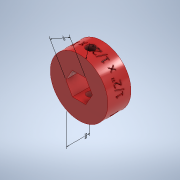
# Autodesk Inventor part: 1_2x1_2x1-1_2 HexBearing
Saved by Autodesk Inventor 2022.2 (Build 262287000, 287)
## iProperties
Created: 2020-11-08
Part Number: 1_2x1_2x1-1_2 HexBearing
Material: PC/ABS Plastic
Document SubType Name: Modeling
Designer: robst
Density: 0.357273 g/cm^3
Appearance: Red
Author: robst
Autodesk Inventor part; units mm, degrees
ref_plane "YZ Plane" through (0, 0, 0) normal (1, 0, 0) x (0, 1, 0)
ref_plane "XZ Plane" through (0, 0, 0) normal (0, 1, 0) x (-1, 0, 0)
ref_plane "XY Plane" through (0, 0, 0) normal (0, 0, 1) x (1, 0, 0)
sketch "Sketch1" plane through (0, 0, 0) normal (0, 0, 1) x (1, 0, 0)
  line L0 (3.6662, 6.35) -> (7.3323, 0)
  line L1 (7.3323, 0) -> (3.6662, -6.35)
  line L2 (3.6662, -6.35) -> (-3.6662, -6.35)
  line L3 (-3.6662, -6.35) -> (-7.3323, 0)
  line L4 (-7.3323, 0) -> (-3.6662, 6.35)
  line L5 (-3.6662, 6.35) -> (3.6662, 6.35)
  circle A0 centre (0, 0) radius 15.875
  circle A1 centre (0, 0) radius 7.3323 construction
  dimension "d0" = 12.7
  dimension "d2" = 31.75
  dimension "d3" = 8.5427
  constraints: 12 end point, 3 coincident, 1 centre point, 1 horizontal, 1 horizontal alignment, 15 other
  measures "d0" distance between parallel lines of L2 L5
  measures "d2" diameter of A0
extrude "Extrusion1" add sketch "Sketch1" against normal blind 12.7
ref_plane "Work Plane1" through (0, 15.875, 0) normal (0, 1, 0) x (-1, 0, 0)
sketch "Sketch2" plane through (0, 15.875, 0) normal (0, 1, 0) x (-1, 0, 0)
  line L0 (0, -6.35) -> (-25.4, -6.35) construction
  line L1 (15.875, 0) -> (-15.875, 0) construction
  line L2 (-22.9639, -8.255) -> (-24.8226, -8.255)
  line L3 (-24.8226, -8.255) -> (-24.8226, -7.866)
  line L4 (-24.8226, -7.866) -> (-24.131, -7.866)
  line L5 (-24.131, -7.866) -> (-24.131, -5.3126)
  line L6 (-24.131, -5.3126) -> (-24.8226, -5.3126)
  line L7 (-24.8226, -5.3126) -> (-24.8226, -4.9637)
  spline S0 degree 2 poles (-24.8226, -4.9637) (-24.4305, -4.9637) (-24.06, -4.7414) (-24.0353, -4.4326) knots 0 0 0 1 2 2 2
  line L8 (-24.0353, -4.4326) -> (-23.6401, -4.4326)
  line L9 (-23.6401, -4.4326) -> (-23.6401, -7.866)
  line L10 (-23.6401, -7.866) -> (-22.9639, -7.866)
  line L11 (-22.9639, -7.866) -> (-22.9639, -8.255)
  line L12 (-20.6792, -4.2752) -> (-22.1705, -9.0825)
  line L13 (-22.1705, -9.0825) -> (-22.6027, -9.0825)
  line L14 (-22.6027, -9.0825) -> (-21.1176, -4.2752)
  line L15 (-21.1176, -4.2752) -> (-20.6792, -4.2752)
  line L16 (-17.9097, -8.255) -> (-20.2593, -8.255)
  line L17 (-20.2593, -8.255) -> (-20.2593, -7.7147)
  spline S1 degree 2 poles (-20.2593, -7.7147) (-20.0061, -7.4769) (-19.5553, -7.0354) (-19.3392, -6.7977) knots 0 0 0 1 2 2 2
  spline S2 degree 2 poles (-19.3392, -6.7977) (-18.9039, -6.3191) (-18.5858, -5.7448) (-18.5858, -5.4392) knots 0 0 0 1 2 2 2
  spline S3 degree 2 poles (-18.5858, -5.4392) (-18.5858, -5.2786) (-18.6846, -5.0378) (-18.7742, -4.9606) knots 0 0 0 1 2 2 2
  spline S4 degree 2 poles (-18.7742, -4.9606) (-18.8637, -4.8834) (-19.0984, -4.8062) (-19.2404, -4.8062) knots 0 0 0 1 2 2 2
  spline S5 degree 2 poles (-19.2404, -4.8062) (-19.3762, -4.8062) (-19.6541, -4.8742) (-19.7807, -4.9267) knots 0 0 0 1 2 2 2
  spline S6 degree 2 poles (-19.7807, -4.9267) (-19.8888, -4.9699) (-20.0895, -5.0934) (-20.1512, -5.1366) knots 0 0 0 1 2 2 2
  line L18 (-20.1512, -5.1366) -> (-20.179, -5.1366)
  line L19 (-20.179, -5.1366) -> (-20.179, -4.5932)
  spline S7 degree 2 poles (-20.179, -4.5932) (-20.0215, -4.516) (-19.4565, -4.3647) (-19.2033, -4.3647) knots 0 0 0 1 2 2 2
  spline S8 degree 2 poles (-19.2033, -4.3647) (-18.6692, -4.3647) (-18.0671, -4.9297) (-18.0671, -5.4114) knots 0 0 0 1 2 2 2
  spline S9 degree 2 poles (-18.0671, -5.4114) (-18.0671, -5.6368) (-18.1721, -6.0135) (-18.2647, -6.174) knots 0 0 0 1 2 2 2
  spline S10 degree 2 poles (-18.2647, -6.174) (-18.3574, -6.3407) (-18.626, -6.668) (-18.7742, -6.8255) knots 0 0 0 1 2 2 2
  spline S11 degree 2 poles (-18.7742, -6.8255) (-19.015, -7.0879) (-19.6047, -7.6498) (-19.7807, -7.8135) knots 0 0 0 1 2 2 2
  line L20 (-19.7807, -7.8135) -> (-17.9097, -7.8135)
  line L21 (-17.9097, -7.8135) -> (-17.9097, -8.255)
  line L22 (-15.8657, -4.2752) -> (-15.9769, -5.7572)
  line L23 (-15.9769, -5.7572) -> (-16.3134, -5.7572)
  line L24 (-16.3134, -5.7572) -> (-16.4246, -4.2752)
  line L25 (-16.4246, -4.2752) -> (-15.8657, -4.2752)
  line L26 (-16.829, -4.2752) -> (-16.9402, -5.7572)
  line L27 (-16.9402, -5.7572) -> (-17.2767, -5.7572)
  line L28 (-17.2767, -5.7572) -> (-17.3879, -4.2752)
  line L29 (-17.3879, -4.2752) -> (-16.829, -4.2752)
  line L30 (-11.3703, -8.255) -> (-11.96, -8.255)
  line L31 (-11.96, -8.255) -> (-12.6547, -7.1805)
  line L32 (-12.6547, -7.1805) -> (-13.3679, -8.255)
  line L33 (-13.3679, -8.255) -> (-13.9144, -8.255)
  line L34 (-13.9144, -8.255) -> (-12.9233, -6.8378)
  line L35 (-12.9233, -6.8378) -> (-13.9052, -5.396)
  line L36 (-13.9052, -5.396) -> (-13.3154, -5.396)
  line L37 (-13.3154, -5.396) -> (-12.6238, -6.4612)
  line L38 (-12.6238, -6.4612) -> (-11.9168, -5.396)
  line L39 (-11.9168, -5.396) -> (-11.3703, -5.396)
  line L40 (-11.3703, -5.396) -> (-12.3552, -6.807)
  line L41 (-12.3552, -6.807) -> (-11.3703, -8.255)
  line L42 (-7.2732, -8.255) -> (-9.1319, -8.255)
  line L43 (-9.1319, -8.255) -> (-9.1319, -7.866)
  line L44 (-9.1319, -7.866) -> (-8.4403, -7.866)
  line L45 (-8.4403, -7.866) -> (-8.4403, -5.3126)
  line L46 (-8.4403, -5.3126) -> (-9.1319, -5.3126)
  line L47 (-9.1319, -5.3126) -> (-9.1319, -4.9637)
  spline S12 degree 2 poles (-9.1319, -4.9637) (-8.7397, -4.9637) (-8.3692, -4.7414) (-8.3445, -4.4326) knots 0 0 0 1 2 2 2
  line L48 (-8.3445, -4.4326) -> (-7.9493, -4.4326)
  line L49 (-7.9493, -4.4326) -> (-7.9493, -7.866)
  line L50 (-7.9493, -7.866) -> (-7.2732, -7.866)
  line L51 (-7.2732, -7.866) -> (-7.2732, -8.255)
  line L52 (-4.9884, -4.2752) -> (-6.4797, -9.0825)
  line L53 (-6.4797, -9.0825) -> (-6.9119, -9.0825)
  line L54 (-6.9119, -9.0825) -> (-5.4268, -4.2752)
  line L55 (-5.4268, -4.2752) -> (-4.9884, -4.2752)
  line L56 (-2.2189, -8.255) -> (-4.5685, -8.255)
  line L57 (-4.5685, -8.255) -> (-4.5685, -7.7147)
  spline S13 degree 2 poles (-4.5685, -7.7147) (-4.3153, -7.4769) (-3.8645, -7.0354) (-3.6484, -6.7977) knots 0 0 0 1 2 2 2
  spline S14 degree 2 poles (-3.6484, -6.7977) (-3.2131, -6.3191) (-2.8951, -5.7448) (-2.8951, -5.4392) knots 0 0 0 1 2 2 2
  spline S15 degree 2 poles (-2.8951, -5.4392) (-2.8951, -5.2786) (-2.9939, -5.0378) (-3.0834, -4.9606) knots 0 0 0 1 2 2 2
  spline S16 degree 2 poles (-3.0834, -4.9606) (-3.1729, -4.8834) (-3.4076, -4.8062) (-3.5496, -4.8062) knots 0 0 0 1 2 2 2
  spline S17 degree 2 poles (-3.5496, -4.8062) (-3.6855, -4.8062) (-3.9633, -4.8742) (-4.0899, -4.9267) knots 0 0 0 1 2 2 2
  spline S18 degree 2 poles (-4.0899, -4.9267) (-4.198, -4.9699) (-4.3987, -5.0934) (-4.4604, -5.1366) knots 0 0 0 1 2 2 2
  line L58 (-4.4604, -5.1366) -> (-4.4882, -5.1366)
  line L59 (-4.4882, -5.1366) -> (-4.4882, -4.5932)
  spline S19 degree 2 poles (-4.4882, -4.5932) (-4.3308, -4.516) (-3.7657, -4.3647) (-3.5126, -4.3647) knots 0 0 0 1 2 2 2
  spline S20 degree 2 poles (-3.5126, -4.3647) (-2.9784, -4.3647) (-2.3764, -4.9297) (-2.3764, -5.4114) knots 0 0 0 1 2 2 2
  spline S21 degree 2 poles (-2.3764, -5.4114) (-2.3764, -5.6368) (-2.4813, -6.0135) (-2.574, -6.174) knots 0 0 0 1 2 2 2
  spline S22 degree 2 poles (-2.574, -6.174) (-2.6666, -6.3407) (-2.9352, -6.668) (-3.0834, -6.8255) knots 0 0 0 1 2 2 2
  spline S23 degree 2 poles (-3.0834, -6.8255) (-3.3242, -7.0879) (-3.9139, -7.6498) (-4.0899, -7.8135) knots 0 0 0 1 2 2 2
  line L60 (-4.0899, -7.8135) -> (-2.2189, -7.8135)
  line L61 (-2.2189, -7.8135) -> (-2.2189, -8.255)
  line L62 (-0.175, -4.2752) -> (-0.2861, -5.7572)
  line L63 (-0.2861, -5.7572) -> (-0.6226, -5.7572)
  line L64 (-0.6226, -5.7572) -> (-0.7338, -4.2752)
  line L65 (-0.7338, -4.2752) -> (-0.175, -4.2752)
  line L66 (-1.1383, -4.2752) -> (-1.2494, -5.7572)
  line L67 (-1.2494, -5.7572) -> (-1.586, -5.7572)
  line L68 (-1.586, -5.7572) -> (-1.6971, -4.2752)
  line L69 (-1.6971, -4.2752) -> (-1.1383, -4.2752)
  line L70 (5.9569, -8.255) -> (5.3671, -8.255)
  line L71 (5.3671, -8.255) -> (4.6724, -7.1805)
  line L72 (4.6724, -7.1805) -> (3.9592, -8.255)
  line L73 (3.9592, -8.255) -> (3.4127, -8.255)
  line L74 (3.4127, -8.255) -> (4.4038, -6.8378)
  line L75 (4.4038, -6.8378) -> (3.422, -5.396)
  line L76 (3.422, -5.396) -> (4.0117, -5.396)
  line L77 (4.0117, -5.396) -> (4.7033, -6.4612)
  line L78 (4.7033, -6.4612) -> (5.4104, -5.396)
  line L79 (5.4104, -5.396) -> (5.9569, -5.396)
  line L80 (5.9569, -5.396) -> (4.9719, -6.807)
  line L81 (4.9719, -6.807) -> (5.9569, -8.255)
  line L82 (10.054, -8.255) -> (8.1953, -8.255)
  line L83 (8.1953, -8.255) -> (8.1953, -7.866)
  line L84 (8.1953, -7.866) -> (8.8869, -7.866)
  line L85 (8.8869, -7.866) -> (8.8869, -5.3126)
  line L86 (8.8869, -5.3126) -> (8.1953, -5.3126)
  line L87 (8.1953, -5.3126) -> (8.1953, -4.9637)
  spline S24 degree 2 poles (8.1953, -4.9637) (8.5874, -4.9637) (8.9579, -4.7414) (8.9826, -4.4326) knots 0 0 0 1 2 2 2
  line L88 (8.9826, -4.4326) -> (9.3778, -4.4326)
  line L89 (9.3778, -4.4326) -> (9.3778, -7.866)
  line L90 (9.3778, -7.866) -> (10.054, -7.866)
  line L91 (10.054, -7.866) -> (10.054, -8.255)
  line L92 (14.5494, -8.255) -> (12.6907, -8.255)
  line L93 (12.6907, -8.255) -> (12.6907, -7.866)
  line L94 (12.6907, -7.866) -> (13.3823, -7.866)
  line L95 (13.3823, -7.866) -> (13.3823, -5.3126)
  line L96 (13.3823, -5.3126) -> (12.6907, -5.3126)
  line L97 (12.6907, -5.3126) -> (12.6907, -4.9637)
  spline S25 degree 2 poles (12.6907, -4.9637) (13.0829, -4.9637) (13.4534, -4.7414) (13.4781, -4.4326) knots 0 0 0 1 2 2 2
  line L98 (13.4781, -4.4326) -> (13.8733, -4.4326)
  line L99 (13.8733, -4.4326) -> (13.8733, -7.866)
  line L100 (13.8733, -7.866) -> (14.5494, -7.866)
  line L101 (14.5494, -7.866) -> (14.5494, -8.255)
  line L102 (16.8342, -4.2752) -> (15.3429, -9.0825)
  line L103 (15.3429, -9.0825) -> (14.9107, -9.0825)
  line L104 (14.9107, -9.0825) -> (16.3958, -4.2752)
  line L105 (16.3958, -4.2752) -> (16.8342, -4.2752)
  line L106 (19.6037, -8.255) -> (17.2541, -8.255)
  line L107 (17.2541, -8.255) -> (17.2541, -7.7147)
  spline S26 degree 2 poles (17.2541, -7.7147) (17.5073, -7.4769) (17.958, -7.0354) (18.1742, -6.7977) knots 0 0 0 1 2 2 2
  spline S27 degree 2 poles (18.1742, -6.7977) (18.6095, -6.3191) (18.9275, -5.7448) (18.9275, -5.4392) knots 0 0 0 1 2 2 2
  spline S28 degree 2 poles (18.9275, -5.4392) (18.9275, -5.2786) (18.8287, -5.0378) (18.7392, -4.9606) knots 0 0 0 1 2 2 2
  spline S29 degree 2 poles (18.7392, -4.9606) (18.6497, -4.8834) (18.415, -4.8062) (18.273, -4.8062) knots 0 0 0 1 2 2 2
  spline S30 degree 2 poles (18.273, -4.8062) (18.1371, -4.8062) (17.8592, -4.8742) (17.7327, -4.9267) knots 0 0 0 1 2 2 2
  spline S31 degree 2 poles (17.7327, -4.9267) (17.6246, -4.9699) (17.4239, -5.0934) (17.3622, -5.1366) knots 0 0 0 1 2 2 2
  line L108 (17.3622, -5.1366) -> (17.3344, -5.1366)
  line L109 (17.3344, -5.1366) -> (17.3344, -4.5932)
  spline S32 degree 2 poles (17.3344, -4.5932) (17.4918, -4.516) (18.0568, -4.3647) (18.31, -4.3647) knots 0 0 0 1 2 2 2
  spline S33 degree 2 poles (18.31, -4.3647) (18.8442, -4.3647) (19.4462, -4.9297) (19.4462, -5.4114) knots 0 0 0 1 2 2 2
  spline S34 degree 2 poles (19.4462, -5.4114) (19.4462, -5.6368) (19.3413, -6.0135) (19.2486, -6.174) knots 0 0 0 1 2 2 2
  spline S35 degree 2 poles (19.2486, -6.174) (19.156, -6.3407) (18.8874, -6.668) (18.7392, -6.8255) knots 0 0 0 1 2 2 2
  spline S36 degree 2 poles (18.7392, -6.8255) (18.4984, -7.0879) (17.9086, -7.6498) (17.7327, -7.8135) knots 0 0 0 1 2 2 2
  line L110 (17.7327, -7.8135) -> (19.6037, -7.8135)
  line L111 (19.6037, -7.8135) -> (19.6037, -8.255)
  line L112 (21.6476, -4.2752) -> (21.5365, -5.7572)
  line L113 (21.5365, -5.7572) -> (21.1999, -5.7572)
  line L114 (21.1999, -5.7572) -> (21.0888, -4.2752)
  line L115 (21.0888, -4.2752) -> (21.6476, -4.2752)
  line L116 (20.6843, -4.2752) -> (20.5732, -5.7572)
  line L117 (20.5732, -5.7572) -> (20.2366, -5.7572)
  line L118 (20.2366, -5.7572) -> (20.1255, -4.2752)
  line L119 (20.1255, -4.2752) -> (20.6843, -4.2752)
  line L120 (27.8041, -8.255) -> (27.3225, -8.255)
  line L121 (27.3225, -8.255) -> (27.3225, -6.6248)
  spline S37 degree 2 poles (27.3225, -6.6248) (27.3225, -6.4272) (27.2854, -6.0876) (27.2299, -5.9857) knots 0 0 0 1 2 2 2
  spline S38 degree 2 poles (27.2299, -5.9857) (27.1712, -5.8776) (26.9613, -5.7726) (26.7822, -5.7726) knots 0 0 0 1 2 2 2
  spline S39 degree 2 poles (26.7822, -5.7726) (26.6031, -5.7726) (26.2233, -5.9641) (26.0412, -6.1184) knots 0 0 0 1 2 2 2
  line L122 (26.0412, -6.1184) -> (26.0412, -8.255)
  line L123 (26.0412, -8.255) -> (25.5595, -8.255)
  line L124 (25.5595, -8.255) -> (25.5595, -4.2752)
  line L125 (25.5595, -4.2752) -> (26.0412, -4.2752)
  line L126 (26.0412, -4.2752) -> (26.0412, -5.714)
  spline S40 degree 2 poles (26.0412, -5.714) (26.2573, -5.5195) (26.6741, -5.3157) (26.9088, -5.3157) knots 0 0 0 1 2 2 2
  spline S41 degree 2 poles (26.9088, -5.3157) (27.3287, -5.3157) (27.8041, -5.8714) (27.8041, -6.3994) knots 0 0 0 1 2 2 2
  line L127 (27.8041, -6.3994) -> (27.8041, -8.255)
  spline S42 degree 2 poles (29.7215, -8.3198) (29.0361, -8.3198) (28.2827, -7.551) (28.2827, -6.8409) knots 0 0 0 1 2 2 2
  spline S43 degree 2 poles (28.2827, -6.8409) (28.2827, -6.1431) (29.0145, -5.3157) (29.6042, -5.3157) knots 0 0 0 1 2 2 2
  spline S44 degree 2 poles (29.6042, -5.3157) (29.8697, -5.3157) (30.2803, -5.4701) (30.4316, -5.6337) knots 0 0 0 1 2 2 2
  spline S45 degree 2 poles (30.4316, -5.6337) (30.586, -5.7973) (30.7496, -6.2697) (30.7496, -6.6124) knots 0 0 0 1 2 2 2
  line L128 (30.7496, -6.6124) -> (30.7496, -6.8749)
  line L129 (30.7496, -6.8749) -> (28.7705, -6.8749)
  spline S46 degree 2 poles (28.7705, -6.8749) (28.7705, -7.372) (29.2707, -7.8999) (29.7153, -7.8999) knots 0 0 0 1 2 2 2
  spline S47 degree 2 poles (29.7153, -7.8999) (29.8728, -7.8999) (30.1785, -7.8289) (30.302, -7.7733) knots 0 0 0 1 2 2 2
  spline S48 degree 2 poles (30.302, -7.7733) (30.4316, -7.7116) (30.6107, -7.6035) (30.6694, -7.5541) knots 0 0 0 1 2 2 2
  line L130 (30.6694, -7.5541) -> (30.6972, -7.5541)
  line L131 (30.6972, -7.5541) -> (30.6972, -8.079)
  spline S49 degree 2 poles (30.6972, -8.079) (30.6138, -8.113) (30.3606, -8.2118) (30.2618, -8.2396) knots 0 0 0 1 2 2 2
  spline S50 degree 2 poles (30.2618, -8.2396) (30.1229, -8.2797) (29.8944, -8.3198) (29.7215, -8.3198) knots 0 0 0 1 2 2 2
  spline S51 degree 2 poles (30.2803, -6.5075) (30.2742, -6.3129) (30.1939, -6.0289) (30.1167, -5.9332) knots 0 0 0 1 2 2 2
  spline S52 degree 2 poles (30.1167, -5.9332) (30.0333, -5.8251) (29.7709, -5.7109) (29.5764, -5.7109) knots 0 0 0 1 2 2 2
  spline S53 degree 2 poles (29.5764, -5.7109) (29.385, -5.7109) (29.1163, -5.8251) (29.0052, -5.9363) knots 0 0 0 1 2 2 2
  spline S54 degree 2 poles (29.0052, -5.9363) (28.8971, -6.0505) (28.786, -6.3253) (28.7705, -6.5075) knots 0 0 0 1 2 2 2
  line L132 (28.7705, -6.5075) -> (30.2803, -6.5075)
  line L133 (33.4574, -8.255) -> (32.8677, -8.255)
  line L134 (32.8677, -8.255) -> (32.173, -7.1805)
  line L135 (32.173, -7.1805) -> (31.4598, -8.255)
  line L136 (31.4598, -8.255) -> (30.9133, -8.255)
  line L137 (30.9133, -8.255) -> (31.9044, -6.8378)
  line L138 (31.9044, -6.8378) -> (30.9225, -5.396)
  line L139 (30.9225, -5.396) -> (31.5123, -5.396)
  line L140 (31.5123, -5.396) -> (32.2039, -6.4612)
  line L141 (32.2039, -6.4612) -> (32.9109, -5.396)
  line L142 (32.9109, -5.396) -> (33.4574, -5.396)
  line L143 (33.4574, -5.396) -> (32.4725, -6.807)
  line L144 (32.4725, -6.807) -> (33.4574, -8.255)
  spline S55 degree 2 poles (37.8633, -6.7792) (37.8633, -7.48) (37.184, -8.3353) (36.6715, -8.3353) knots 0 0 0 1 2 2 2
  spline S56 degree 2 poles (36.6715, -8.3353) (36.4399, -8.3353) (36.1096, -8.221) (35.949, -8.1222) knots 0 0 0 1 2 2 2
  line L145 (35.949, -8.1222) -> (35.9182, -8.255)
  line L146 (35.9182, -8.255) -> (35.4674, -8.255)
  line L147 (35.4674, -8.255) -> (35.4674, -4.2752)
  line L148 (35.4674, -4.2752) -> (35.949, -4.2752)
  line L149 (35.949, -4.2752) -> (35.949, -5.6954)
  spline S57 degree 2 poles (35.949, -5.6954) (36.1312, -5.5318) (36.5542, -5.3157) (36.8228, -5.3157) knots 0 0 0 1 2 2 2
  spline S58 degree 2 poles (36.8228, -5.3157) (37.3075, -5.3157) (37.8633, -6.0906) (37.8633, -6.7792) knots 0 0 0 1 2 2 2
  spline S59 degree 2 poles (37.3662, -6.8162) (37.3662, -6.3037) (37.0544, -5.7726) (36.7086, -5.7726) knots 0 0 0 1 2 2 2
  spline S60 degree 2 poles (36.7086, -5.7726) (36.514, -5.7726) (36.1127, -5.9579) (35.949, -6.0999) knots 0 0 0 1 2 2 2
  line L150 (35.949, -6.0999) -> (35.949, -7.7394)
  spline S61 degree 2 poles (35.949, -7.7394) (36.1312, -7.8289) (36.4122, -7.903) (36.5789, -7.903) knots 0 0 0 1 2 2 2
  spline S62 degree 2 poles (36.5789, -7.903) (36.9463, -7.903) (37.3662, -7.3812) (37.3662, -6.8162) knots 0 0 0 1 2 2 2
  line L151 (40.5865, -8.255) -> (40.1048, -8.255)
  line L152 (40.1048, -8.255) -> (40.1048, -7.9401)
  spline S63 degree 2 poles (40.1048, -7.9401) (39.8825, -8.1346) (39.4842, -8.3353) (39.2372, -8.3353) knots 0 0 0 1 2 2 2
  spline S64 degree 2 poles (39.2372, -8.3353) (39.052, -8.3353) (38.7216, -8.2118) (38.6012, -8.079) knots 0 0 0 1 2 2 2
  spline S65 degree 2 poles (38.6012, -8.079) (38.4777, -7.9462) (38.3419, -7.5418) (38.3419, -7.2516) knots 0 0 0 1 2 2 2
  line L153 (38.3419, -7.2516) -> (38.3419, -5.396)
  line L154 (38.3419, -5.396) -> (38.8235, -5.396)
  line L155 (38.8235, -5.396) -> (38.8235, -7.0262)
  spline S66 degree 2 poles (38.8235, -7.0262) (38.8235, -7.2546) (38.8575, -7.5541) (38.9161, -7.6653) knots 0 0 0 1 2 2 2
  spline S67 degree 2 poles (38.9161, -7.6653) (38.9748, -7.7764) (39.1755, -7.8783) (39.3638, -7.8783) knots 0 0 0 1 2 2 2
  spline S68 degree 2 poles (39.3638, -7.8783) (39.5398, -7.8783) (39.9381, -7.6776) (40.1048, -7.5325) knots 0 0 0 1 2 2 2
  line L156 (40.1048, -7.5325) -> (40.1048, -5.396)
  line L157 (40.1048, -5.396) -> (40.5865, -5.396)
  line L158 (40.5865, -5.396) -> (40.5865, -8.255)
  spline S69 degree 2 poles (42.0561, -8.3229) (41.769, -8.3229) (41.2719, -8.1685) (41.1083, -8.0821) knots 0 0 0 1 2 2 2
  line L159 (41.1083, -8.0821) -> (41.1083, -7.5418)
  line L160 (41.1083, -7.5418) -> (41.133, -7.5418)
  spline S70 degree 2 poles (41.133, -7.5418) (41.1947, -7.5912) (41.3615, -7.7085) (41.5004, -7.7733) knots 0 0 0 1 2 2 2
  spline S71 degree 2 poles (41.5004, -7.7733) (41.6208, -7.832) (41.9172, -7.9185) (42.0747, -7.9185) knots 0 0 0 1 2 2 2
  spline S72 degree 2 poles (42.0747, -7.9185) (42.1889, -7.9185) (42.4513, -7.866) (42.5131, -7.8227) knots 0 0 0 1 2 2 2
  spline S73 degree 2 poles (42.5131, -7.8227) (42.6026, -7.7641) (42.6829, -7.6313) (42.6829, -7.4955) knots 0 0 0 1 2 2 2
  spline S74 degree 2 poles (42.6829, -7.4955) (42.6829, -7.3257) (42.4977, -7.1497) (42.2599, -7.091) knots 0 0 0 1 2 2 2
  spline S75 degree 2 poles (42.2599, -7.091) (42.1673, -7.0694) (41.8709, -7.0076) (41.7443, -6.9737) knots 0 0 0 1 2 2 2
  spline S76 degree 2 poles (41.7443, -6.9737) (41.417, -6.878) (41.1206, -6.4828) (41.1206, -6.2018) knots 0 0 0 1 2 2 2
  spline S77 degree 2 poles (41.1206, -6.2018) (41.1206, -5.8128) (41.7042, -5.328) (42.1858, -5.328) knots 0 0 0 1 2 2 2
  spline S78 degree 2 poles (42.1858, -5.328) (42.4236, -5.328) (42.9052, -5.4454) (43.0689, -5.5349) knots 0 0 0 1 2 2 2
  line L161 (43.0689, -5.5349) -> (43.0689, -6.0505)
  line L162 (43.0689, -6.0505) -> (43.0442, -6.0505)
  spline S79 degree 2 poles (43.0442, -6.0505) (42.8589, -5.9023) (42.4081, -5.7325) (42.1766, -5.7325) knots 0 0 0 1 2 2 2
  spline S80 degree 2 poles (42.1766, -5.7325) (41.9388, -5.7325) (41.6115, -5.9332) (41.6115, -6.1339) knots 0 0 0 1 2 2 2
  spline S81 degree 2 poles (41.6115, -6.1339) (41.6115, -6.316) (41.8061, -6.492) (42.0222, -6.5476) knots 0 0 0 1 2 2 2
  spline S82 degree 2 poles (42.0222, -6.5476) (42.1272, -6.5754) (42.3927, -6.631) (42.5378, -6.6649) knots 0 0 0 1 2 2 2
  spline S83 degree 2 poles (42.5378, -6.6649) (42.8527, -6.7452) (43.1738, -7.1126) (43.1738, -7.4306) knots 0 0 0 1 2 2 2
  spline S84 degree 2 poles (43.1738, -7.4306) (43.1738, -7.6159) (43.0287, -7.9432) (42.8867, -8.0636) knots 0 0 0 1 2 2 2
  spline S85 degree 2 poles (42.8867, -8.0636) (42.7354, -8.1902) (42.3495, -8.3229) (42.0561, -8.3229) knots 0 0 0 1 2 2 2
  line L163 (45.8661, -8.255) -> (45.3845, -8.255)
  line L164 (45.3845, -8.255) -> (45.3845, -6.6248)
  spline S86 degree 2 poles (45.3845, -6.6248) (45.3845, -6.4272) (45.3474, -6.0876) (45.2919, -5.9857) knots 0 0 0 1 2 2 2
  spline S87 degree 2 poles (45.2919, -5.9857) (45.2332, -5.8776) (45.0233, -5.7726) (44.8442, -5.7726) knots 0 0 0 1 2 2 2
  spline S88 degree 2 poles (44.8442, -5.7726) (44.6651, -5.7726) (44.2853, -5.9641) (44.1032, -6.1184) knots 0 0 0 1 2 2 2
  line L165 (44.1032, -6.1184) -> (44.1032, -8.255)
  line L166 (44.1032, -8.255) -> (43.6215, -8.255)
  line L167 (43.6215, -8.255) -> (43.6215, -4.2752)
  line L168 (43.6215, -4.2752) -> (44.1032, -4.2752)
  line L169 (44.1032, -4.2752) -> (44.1032, -5.714)
  spline S89 degree 2 poles (44.1032, -5.714) (44.3193, -5.5195) (44.7361, -5.3157) (44.9708, -5.3157) knots 0 0 0 1 2 2 2
  spline S90 degree 2 poles (44.9708, -5.3157) (45.3907, -5.3157) (45.8661, -5.8714) (45.8661, -6.3994) knots 0 0 0 1 2 2 2
  line L170 (45.8661, -6.3994) -> (45.8661, -8.255)
  line L171 (47.0332, -8.255) -> (46.5516, -8.255)
  line L172 (46.5516, -8.255) -> (46.5516, -5.396)
  line L173 (46.5516, -5.396) -> (47.0332, -5.396)
  line L174 (47.0332, -5.396) -> (47.0332, -8.255)
  line L175 (47.0672, -4.9205) -> (46.5207, -4.9205)
  line L176 (46.5207, -4.9205) -> (46.5207, -4.4203)
  line L177 (46.5207, -4.4203) -> (47.0672, -4.4203)
  line L178 (47.0672, -4.4203) -> (47.0672, -4.9205)
  line L179 (49.9849, -8.255) -> (49.5032, -8.255)
  line L180 (49.5032, -8.255) -> (49.5032, -6.6248)
  spline S91 degree 2 poles (49.5032, -6.6248) (49.5032, -6.4272) (49.4662, -6.0876) (49.4106, -5.9857) knots 0 0 0 1 2 2 2
  spline S92 degree 2 poles (49.4106, -5.9857) (49.352, -5.8776) (49.142, -5.7726) (48.9629, -5.7726) knots 0 0 0 1 2 2 2
  spline S93 degree 2 poles (48.9629, -5.7726) (48.7839, -5.7726) (48.4041, -5.9641) (48.2219, -6.1184) knots 0 0 0 1 2 2 2
  line L181 (48.2219, -6.1184) -> (48.2219, -8.255)
  line L182 (48.2219, -8.255) -> (47.7403, -8.255)
  line L183 (47.7403, -8.255) -> (47.7403, -5.396)
  line L184 (47.7403, -5.396) -> (48.2219, -5.396)
  line L185 (48.2219, -5.396) -> (48.2219, -5.714)
  spline S94 degree 2 poles (48.2219, -5.714) (48.438, -5.5195) (48.8549, -5.3157) (49.0895, -5.3157) knots 0 0 0 1 2 2 2
  spline S95 degree 2 poles (49.0895, -5.3157) (49.5094, -5.3157) (49.9849, -5.8714) (49.9849, -6.3994) knots 0 0 0 1 2 2 2
  line L186 (49.9849, -6.3994) -> (49.9849, -8.255)
  spline S96 degree 2 poles (50.763, -8.712) (50.8124, -8.7336) (51.0007, -8.8015) (51.1211, -8.8293) knots 0 0 0 1 2 2 2
  spline S97 degree 2 poles (51.1211, -8.8293) (51.2539, -8.8632) (51.4793, -8.9034) (51.612, -8.9034) knots 0 0 0 1 2 2 2
  spline S98 degree 2 poles (51.612, -8.9034) (51.8343, -8.9034) (52.1431, -8.7861) (52.2295, -8.6811) knots 0 0 0 1 2 2 2
  spline S99 degree 2 poles (52.2295, -8.6811) (52.3129, -8.5761) (52.3777, -8.3013) (52.3777, -8.1253) knots 0 0 0 1 2 2 2
  line L187 (52.3777, -8.1253) -> (52.3777, -7.8752)
  spline S100 degree 2 poles (52.3777, -7.8752) (52.1832, -8.045) (51.8096, -8.2056) (51.5287, -8.2056) knots 0 0 0 1 2 2 2
  spline S101 degree 2 poles (51.5287, -8.2056) (51.0408, -8.2056) (50.4635, -7.48) (50.4635, -6.7977) knots 0 0 0 1 2 2 2
  spline S102 degree 2 poles (50.4635, -6.7977) (50.4635, -6.4426) (50.6642, -5.893) (50.8309, -5.6985) knots 0 0 0 1 2 2 2
  spline S103 degree 2 poles (50.8309, -5.6985) (50.9914, -5.5164) (51.4329, -5.3157) (51.6676, -5.3157) knots 0 0 0 1 2 2 2
  spline S104 degree 2 poles (51.6676, -5.3157) (51.8899, -5.3157) (52.2141, -5.4207) (52.3777, -5.5164) knots 0 0 0 1 2 2 2
  line L188 (52.3777, -5.5164) -> (52.4055, -5.396)
  line L189 (52.4055, -5.396) -> (52.8594, -5.396)
  line L190 (52.8594, -5.396) -> (52.8594, -7.9277)
  spline S105 degree 2 poles (52.8594, -7.9277) (52.8594, -8.6564) (52.2264, -9.3356) (51.575, -9.3356) knots 0 0 0 1 2 2 2
  spline S106 degree 2 poles (51.575, -9.3356) (51.365, -9.3356) (50.9266, -9.2677) (50.7383, -9.2121) knots 0 0 0 1 2 2 2
  line L191 (50.7383, -9.2121) -> (50.7383, -8.712)
  line L192 (50.7383, -8.712) -> (50.763, -8.712)
  line L193 (52.3777, -7.48) -> (52.3777, -5.9085)
  spline S107 degree 2 poles (52.3777, -5.9085) (52.1986, -5.822) (51.8961, -5.7479) (51.7448, -5.7479) knots 0 0 0 1 2 2 2
  spline S108 degree 2 poles (51.7448, -5.7479) (51.3805, -5.7479) (50.9606, -6.2852) (50.9606, -6.7884) knots 0 0 0 1 2 2 2
  spline S109 degree 2 poles (50.9606, -6.7884) (50.9606, -7.2639) (51.2786, -7.761) (51.6367, -7.761) knots 0 0 0 1 2 2 2
  spline S110 degree 2 poles (51.6367, -7.761) (51.8251, -7.761) (52.2203, -7.6128) (52.3777, -7.48) knots 0 0 0 1 2 2 2
  spline S111 degree 2 poles (57.5895, -6.7483) (57.5895, -7.4646) (56.9071, -8.3106) (56.3853, -8.3106) knots 0 0 0 1 2 2 2
  spline S112 degree 2 poles (56.3853, -8.3106) (56.1723, -8.3106) (55.845, -8.2118) (55.6752, -8.1099) knots 0 0 0 1 2 2 2
  line L194 (55.6752, -8.1099) -> (55.6752, -9.3078)
  line L195 (55.6752, -9.3078) -> (55.1935, -9.3078)
  line L196 (55.1935, -9.3078) -> (55.1935, -5.396)
  line L197 (55.1935, -5.396) -> (55.6752, -5.396)
  line L198 (55.6752, -5.396) -> (55.6752, -5.6954)
  spline S113 degree 2 poles (55.6752, -5.6954) (55.8543, -5.5318) (56.2927, -5.3157) (56.549, -5.3157) knots 0 0 0 1 2 2 2
  spline S114 degree 2 poles (56.549, -5.3157) (57.0399, -5.3157) (57.5895, -6.0937) (57.5895, -6.7483) knots 0 0 0 1 2 2 2
  spline S115 degree 2 poles (57.0924, -6.8039) (57.0924, -6.3129) (56.7805, -5.7726) (56.4316, -5.7726) knots 0 0 0 1 2 2 2
  spline S116 degree 2 poles (56.4316, -5.7726) (56.2279, -5.7726) (55.845, -5.9548) (55.6752, -6.0968) knots 0 0 0 1 2 2 2
  line L199 (55.6752, -6.0968) -> (55.6752, -7.7209)
  spline S117 degree 2 poles (55.6752, -7.7209) (55.8635, -7.8104) (56.1321, -7.8783) (56.305, -7.8783) knots 0 0 0 1 2 2 2
  spline S118 degree 2 poles (56.305, -7.8783) (56.6786, -7.8783) (57.0924, -7.3287) (57.0924, -6.8039) knots 0 0 0 1 2 2 2
  line L200 (60.3343, -5.396) -> (59.2567, -8.255)
  line L201 (59.2567, -8.255) -> (58.8245, -8.255)
  line L202 (58.8245, -8.255) -> (57.7562, -5.396)
  line L203 (57.7562, -5.396) -> (58.278, -5.396)
  line L204 (58.278, -5.396) -> (59.0591, -7.5974)
  line L205 (59.0591, -7.5974) -> (59.8341, -5.396)
  line L206 (59.8341, -5.396) -> (60.3343, -5.396)
  spline S119 degree 2 poles (62.9988, -6.35) (62.9988, -7.3751) (62.4029, -8.3353) (61.7823, -8.3353) knots 0 0 0 1 2 2 2
  spline S120 degree 2 poles (61.7823, -8.3353) (61.1525, -8.3353) (60.5627, -7.3565) (60.5627, -6.3531) knots 0 0 0 1 2 2 2
  spline S121 degree 2 poles (60.5627, -6.3531) (60.5627, -5.3219) (61.1586, -4.3678) (61.7823, -4.3678) knots 0 0 0 1 2 2 2
  spline S122 degree 2 poles (61.7823, -4.3678) (62.4091, -4.3678) (62.9988, -5.3558) (62.9988, -6.35) knots 0 0 0 1 2 2 2
  spline S123 degree 2 poles (62.3442, -7.5109) (62.4183, -7.3226) (62.4801, -6.7421) (62.4801, -6.35) knots 0 0 0 1 2 2 2
  spline S124 degree 2 poles (62.4801, -6.35) (62.4801, -5.9579) (62.4183, -5.3805) (62.3412, -5.186) knots 0 0 0 1 2 2 2
  spline S125 degree 2 poles (62.3412, -5.186) (62.264, -4.9915) (61.9953, -4.7908) (61.7823, -4.7908) knots 0 0 0 1 2 2 2
  spline S126 degree 2 poles (61.7823, -4.7908) (61.5693, -4.7908) (61.2945, -4.9915) (61.2142, -5.1922) knots 0 0 0 1 2 2 2
  spline S127 degree 2 poles (61.2142, -5.1922) (61.137, -5.3867) (61.0814, -5.9795) (61.0814, -6.3531) knots 0 0 0 1 2 2 2
  spline S128 degree 2 poles (61.0814, -6.3531) (61.0814, -6.7545) (61.1308, -7.2917) (61.2111, -7.5016) knots 0 0 0 1 2 2 2
  spline S129 degree 2 poles (61.2111, -7.5016) (61.2852, -7.6992) (61.56, -7.9123) (61.7823, -7.9123) knots 0 0 0 1 2 2 2
  spline S130 degree 2 poles (61.7823, -7.9123) (61.9923, -7.9123) (62.2671, -7.7116) (62.3442, -7.5109) knots 0 0 0 1 2 2 2
  line L207 (65.6448, -8.255) -> (63.7861, -8.255)
  line L208 (63.7861, -8.255) -> (63.7861, -7.866)
  line L209 (63.7861, -7.866) -> (64.4777, -7.866)
  line L210 (64.4777, -7.866) -> (64.4777, -5.3126)
  line L211 (64.4777, -5.3126) -> (63.7861, -5.3126)
  line L212 (63.7861, -5.3126) -> (63.7861, -4.9637)
  spline S131 degree 2 poles (63.7861, -4.9637) (64.1782, -4.9637) (64.5487, -4.7414) (64.5734, -4.4326) knots 0 0 0 1 2 2 2
  line L213 (64.5734, -4.4326) -> (64.9686, -4.4326)
  line L214 (64.9686, -4.4326) -> (64.9686, -7.866)
  line L215 (64.9686, -7.866) -> (65.6448, -7.866)
  line L216 (65.6448, -7.866) -> (65.6448, -8.255)
  point P0 (0, 0)
  dimension "d17" = 25.4
  dimension "d18" = 6.35
  constraints: 2 end point, 2 horizontal
  measures "d17" distance of L0.start L0.end
  measures "d18" distance between parallel lines of L0 L1
emboss "Emboss1" sketch "Sketch2" operation cut depth 2.54 direction (0, -1, 0) wrap yes faces at (15.8235, -1.2774, -8.4667)
sketch "Sketch3" plane through (0, 15.875, 0) normal (0, 1, 0) x (-1, 0, 0)
  line L0 (3.6662, 0) -> (-3.6662, 0) construction
  line L1 (0, 0) -> (0, -12.7) construction
  line L2 (-3.6662, -12.7) -> (3.6662, -12.7) construction
  line L3 (15.875, 0) -> (-15.875, 0) projected
  line L4 (-15.875, -12.7) -> (15.875, -12.7) projected
  point P0 (0, 0)
  point P1 (0, -6.35)
  dimension "d28" = 6.35
  dimension "d29" = 6.35
  constraints: 3 midpoint, 2 end point
  measures "d28" distance from line of L3 point (0, -6.35)
  measures "d29" distance from line of L4 point (0, -6.35)
hole "Hole1" at (0, 15.875, -6.35) direction (0, -1, 0) diameter 4.318 end through all clearance for "Hex Machine Screw" size "#6" standard "Ansi Unified Screw Threads"
sketch "Sketch4" plane through (0, 15.875, 0) normal (0, 1, 0) x (-1, 0, 0)
  circle A0 centre (0, -6.35) radius 2.159 projected
  circle A1 centre (0, -6.35) radius 2.4257
  point P0 (0, 0)
  point P1 (0, -4.445)
  point P2 (2.0138, -5.8255)
  point P3 (2.0136, -7.3829)
  point P4 (1.4342, -8.2178)
  point P5 (-0.3417, -8.7358)
  point P6 (1.6461, -8.001)
  point P7 (1.1668, -8.4205)
  point P8 (1.1668, -4.7875)
  point P9 (1.6461, -5.207)
  point P10 (1.0457, -8.4928)
  point P11 (0.14, -8.7585)
  point P12 (2.125, -6.2226)
  point P13 (-1.8043, -5.4183)
  point P14 (2.1178, -5.93)
  point P15 (0.209, -4.2011)
  point P16 (2.1178, -5.93)
  point P17 (0, -8.763)
  point P18 (0, -4.4768)
  point P19 (0, -8.7948)
  point P20 (-1.5869, -7.8139)
  point P21 (1.9368, -5.396)
  dimension "d30" = 4.8514
  constraints: 1 centre point, 1 coincident, 7 other
  measures "d30" diameter of A1
extrude "Extrusion2" cut sketch "Sketch4" against normal blind 5.5524 contours A0 | A1
ref_plane "Work Plane2" through (0, -15.875, 0) normal (0, 1, 0) x (-1, 0, 0)
sketch "Sketch5" plane through (0, -15.875, 0) normal (0, 1, 0) x (-1, 0, 0)
  circle A0 centre (0, -6.35) radius 2.159 projected
  circle A1 centre (0, -6.35) radius 3.429
  point P0 (0, 0)
  point P1 (0.9744, -4.4234)
  point P2 (1.04, -8.242)
  point P3 (2.1188, -5.9352)
  point P4 (1.525, -7.8783)
  point P5 (2.0006, -7.1617)
  point P6 (2.12, -5.9412)
  dimension "d33" = 6.858
  constraints: 1 centre point, 1 coincident, 1 other
  measures "d33" diameter of A1
extrude "Extrusion3" cut sketch "Sketch5" along normal blind 1.8542 contours A0 | A1
equation "\"d0\" = hexSize"
equation "\"d2\" = externalDiameter"
equation "\"d4\" = thickness"
equation "\"hexSize\" = 12.7"
equation "\"externalDiameter\" = 31.75"
equation "\"thickness\" = 12.7"
body "Solid1"
